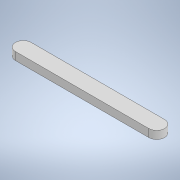
# Autodesk Inventor part: eslabon1
Saved by Autodesk Inventor 2021 (Build 250183000, 183)
## iProperties
Created: 2022-10-24
Part Number: eslabon1
Material: Generic
Document SubType Name: Modeling
Designer: felip
Density: 1 g/cm^3
Appearance: Default
Author: felip
Autodesk Inventor part; units mm, degrees
ref_plane "YZ Plane" through (0, 0, 0) normal (1, 0, 0) x (0, 1, 0)
ref_plane "XZ Plane" through (0, 0, 0) normal (0, 1, 0) x (-1, 0, 0)
ref_plane "XY Plane" through (0, 0, 0) normal (0, 0, 1) x (1, 0, 0)
sketch "Sketch1" plane through (0, 0, 0) normal (0, 1, 0) x (-1, 0, 0)
  line L0 (10, 0) -> (180, 0)
  arc A0 (180, -20) -> (180, 0) centre (180, -10) ccw
  arc A1 (10, 0) -> (10, -20) centre (10, -10) ccw
  line L1 (180, -20) -> (10, -20)
  point P0 (0, 0)
  dimension "d0" = 20
  dimension "d5" = 20
  dimension "d6" = 10
  dimension "d7" = 10
  dimension "d11" = 190
  dimension "d13" = 20
  constraints: 4 end point, 4 point on circle, 2 centre point, 1 horizontal, 1 parallel
  measures "d0" diameter of A0
  measures "d5" diameter of A1
  measures "d6" distance from line of L0 A1.centre
  measures "d7" distance from line of L0 A0.centre
  measures "d13" distance between parallel lines of L0 L1
extrude "Extrusion1" add sketch "Sketch1" along normal blind 10
equation "\"d0\" = d1"
equation "\"d5\" = d0"
equation "\"d6\" = d4"
equation "\"d7\" = 0.5 * d0"
equation "\"d4\" = d3"
equation "\"d1\" = 20"
equation "\"d3\" = 10"
body "Solid1"
